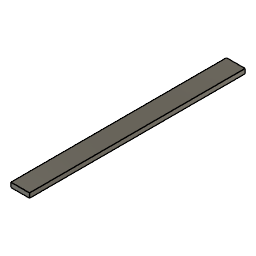
front and back side plates for coil housing (Autodesk Fusion 360 design; units mm, degrees)
part number: 2026-08-05-15-19-59-138
Autodesk Fusion 360 part; units mm, degrees
sketch "Sketch1" plane through (0, 0, 0) normal (0, 0, 1) x (1, 0, 0)
  line L0 (0, 0) -> (25.4, 0)
  line L1 (25.4, 0) -> (25.4, 293.37)
  line L2 (25.4, 293.37) -> (0, 293.37)
  line L3 (0, 293.37) -> (0, 0)
  dimension "d1" = 25.4
  dimension "d2" = 293.37
  constraint horizontal L0
  constraint vertical L1
  constraint horizontal L2
  constraint vertical L3
  constraint coincident L0.start L3.end
  measures "d1" distance of L0.start L0.end
  measures "d2" distance of L0.start L2.end
extrude "Extrude1" add sketch "Sketch1" along normal blind 6.35
